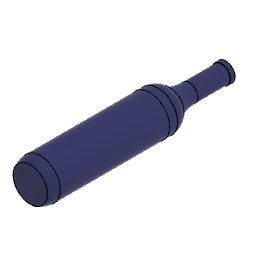
vinflaska v2 (Autodesk Fusion 360 design; units mm, degrees)
Autodesk Fusion 360 part; units mm, degrees
note: some values were not read from the file. Set by a fixed rule: which sketch regions a step uses.
sketch "Sketch1" plane through (0, 0, 0) normal (0, 0, 1) x (1, 0, 0)
  line L0 (0, 0) -> (0, 100.5)
  line L1 (0, 100.5) -> (4.8, 100.5)
  line L2 (4.8, 100.5) -> (4.8, 98.25)
  line L3 (4.8, 98.25) -> (4.5, 98.25)
  line L4 (4.5, 98.25) -> (4.5, 81.7479)
  line L5 (10.2824, 61.4) -> (10.2824, 5.2127)
  line L6 (0, 0) -> (8.8361, 0)
  arc A0 (8.8361, 0) -> (10.2824, 5.2127) centre (0.1654, 5.2127) ccw
  arc A1 (4.5, 81.7479) -> (6.5345, 72.2453) centre (27.709, 81.7479) ccw
  line L7 (10.2054, 65.5631) -> (10.2824, 61.4)
  arc A2 (6.5345, 72.2453) -> (7.5928, 71.4184) centre (7.5928, 72.509) ccw
  arc A3 (10.2054, 65.5631) -> (7.5928, 71.4184) centre (1.998, 65.4114) ccw
  line L8 (8.5816, 71.4184) -> (8.683, 71.4184)
  dimension "d1" = 100.5
  dimension "d2" = 4.8
  dimension "d3" = 2.25
  dimension "d4" = 0.3
  dimension "d5" = 16.5021
  dimension "d13" = 61.4
  constraint coincident L0.start L6.start
  constraint vertical L0
  constraint perpendicular L0 L1
  constraint vertical L2
  constraint horizontal L3
  constraint perpendicular L3 L4
  constraint perpendicular L0 L6
  constraint parallel L0 L5
  constraint tangent L5 A0
  constraint tangent L4 A1
  constraint tangent L7 A3
  measures "d1" distance of L0.start L0.end
  measures "d2" distance of L0.end L1.end
  measures "d3" distance of L1.end L2.end
  measures "d4" distance of L2.end L3.end
  measures "d5" distance of L3.end L4.end
  measures "d13" vertical distance of L5.start L6.end
revolve "Revolve1" add sketch "Sketch1" angle 360 about axis through (0, 0, 0) along (0, 1, 0)
equation "d1 = haed_flosku"
equation "d5 = d1 * 0.1642"
equation "d13 = d1 - 39.1 mm"
equation "haed_flosku = 100.5 mm"
